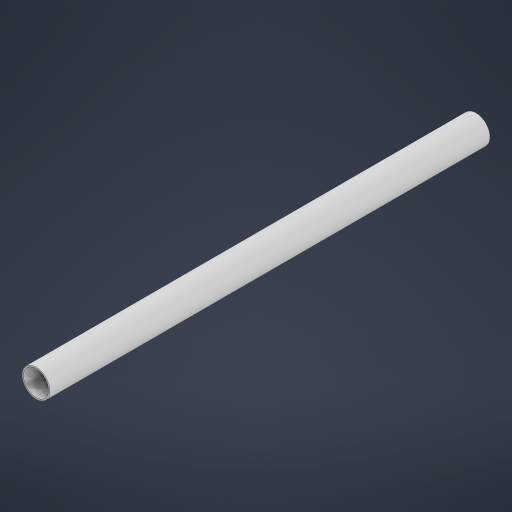
# Autodesk Inventor part: Tubo de 3 mestros
Saved by Autodesk Inventor 2024 (Build 280153000, 153)
## iProperties
Created: 2024-11-05
Part Number: Tubo de 3 mestros
Material: Genérico
Document SubType Name: Modeling
Designer: nesto
Density: 1 g/cm^3
Appearance: Valor por defecto
Author: nesto
Autodesk Inventor part; units mm, degrees
ref_plane "YZ Plane" through (0, 0, 0) normal (1, 0, 0) x (0, 1, 0)
ref_plane "XZ Plane" through (0, 0, 0) normal (0, 1, 0) x (-1, 0, 0)
ref_plane "XY Plane" through (0, 0, 0) normal (0, 0, 1) x (1, 0, 0)
sketch "Boceto1" plane through (0, 0, 0) normal (0, 0, 1) x (1, 0, 0)
  circle A0 centre (0, 0) radius 95
  dimension "d0" = 190
  constraints: 1 centre point, 1 coincident
  measures "d0" diameter of A0
extrude "Extrusión1" add sketch "Boceto1" along normal blind 3000
sketch "Boceto3" plane through (0, 0, 3000) normal (0, 0, 1) x (1, 0, 0)
  circle A0 centre (0, 0) radius 85.31
  dimension "d6" = 170.62
  constraints: 1 centre point, 1 coincident
  measures "d6" diameter of A0
extrude "Extrusión3" cut sketch "Boceto3" against normal blind 3000
